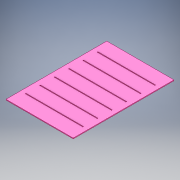
# Autodesk Inventor part: panel
Saved by Autodesk Inventor 2018 (Build 220112000, 112)
## iProperties
Created: 2018-01-24
Part Number: panel
Material: Generic
Document SubType Name: Modeling
Designer: mokuz
Density: 1 g/cm^3
Appearance: Pink
Author: mokuz
Autodesk Inventor part; units mm, degrees
ref_plane "YZ Plane" through (0, 0, 0) normal (1, 0, 0) x (0, 1, 0)
ref_plane "XZ Plane" through (0, 0, 0) normal (0, 1, 0) x (-1, 0, 0)
ref_plane "XY Plane" through (0, 0, 0) normal (0, 0, 1) x (1, 0, 0)
sketch "Sketch1" plane through (0, 0, 0) normal (0, 0, 1) x (1, 0, 0)
  line L0 (0, 0) -> (1400, 0)
  line L1 (1400, 0) -> (1400, 2100)
  line L2 (1400, 2100) -> (0, 2100)
  line L3 (0, 2100) -> (0, 0)
  dimension "d0" = 1400
  dimension "d1" = 2100
  constraints: 8 end point, 2 parallel, 1 horizontal, 1 perpendicular
  measures "d0" distance of L2.end L1.end
  measures "d1" distance of L1.end L0.end
extrude "Extrusion1" add sketch "Sketch1" along normal blind 16
sketch "Sketch2" plane through (0, 0, 16) normal (0, 0, 1) x (1, 0, 0)
  line L0 (1400, 0) -> (1400, 2100) projected
  line L1 (0, 2100) -> (0, 0) projected
  line L2 (0, 0) -> (1400, 0) projected
  line L3 (0, 0) -> (100, 0)
  line L4 (100, 0) -> (100, 300)
  line L5 (100, 300) -> (0, 300)
  line L6 (0, 300) -> (0, 0)
  line L7 (100, 300) -> (1300, 300)
  line L8 (1300, 300) -> (1300, 316)
  line L9 (1300, 316) -> (100, 316)
  line L10 (100, 316) -> (100, 300)
  line L11 (100, 600) -> (1300, 600)
  line L12 (1300, 616) -> (100, 616)
  line L13 (100, 616) -> (100, 600)
  line L14 (1300, 600) -> (1300, 616)
  line L15 (100, 900) -> (1300, 900)
  line L16 (1300, 916) -> (100, 916)
  line L17 (100, 916) -> (100, 900)
  line L18 (1300, 900) -> (1300, 916)
  line L19 (100, 1200) -> (1300, 1200)
  line L20 (1300, 1216) -> (100, 1216)
  line L21 (100, 1216) -> (100, 1200)
  line L22 (1300, 1200) -> (1300, 1216)
  line L23 (100, 1500) -> (1300, 1500)
  line L24 (1300, 1516) -> (100, 1516)
  line L25 (100, 1516) -> (100, 1500)
  line L26 (1300, 1500) -> (1300, 1516)
  line L27 (100, 1800) -> (1300, 1800)
  line L28 (1300, 1816) -> (100, 1816)
  line L29 (100, 1816) -> (100, 1800)
  line L30 (1300, 1800) -> (1300, 1816)
  dimension "d4" = 1400
  dimension "d5" = 100
  dimension "d6" = 300
  dimension "d7" = 1200
  dimension "d8" = 16
  dimension "d13" = 300
  constraints: 56 end point, 4 parallel, 2 horizontal, 2 perpendicular, 1 vertical, 40 other
  measures "d4" distance between parallel lines of L0 L1
  measures "d5" distance of L5.end L4.end
  measures "d6" distance of L4.end L3.end
  measures "d7" distance of L9.end L8.end
  measures "d8" distance of L8.end L7.end
  measures "d13" distance of L4.end L11.start
extrude "Extrusion2" cut sketch "Sketch2" against normal blind 16 contours L10 L9 L8 L7 | L13 L12 L14 L11 | L17 L16 L18 L15 | L21 L20 L22 L19 | L25 L24 L26 L23 | L29 L28 L30 L27
body "Solid1"
